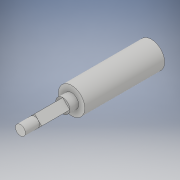
# Autodesk Inventor part: MainGearShaft
Saved by Autodesk Inventor 2017 (Build 210142000, 142)
## iProperties
Created: 2020-04-04
Part Number: MainGearShaft
Material: Generic
Document SubType Name: Modeling
Designer: LaNave
Density: 1 g/cm^3
Appearance: Default
Mass: 3.54669 g
Surface Area: 26.9064 cm^2
Volume: 3.54669 cm^3
Author: LaNave
## iProperties of the stored document gear1-shaft_3DPrint.ipt
Created: 2021-01-25
Part Number: gear1-shaft_3DPrint
Material: Generic
Document SubType Name: Modeling
Designer: agustin
Density: 1 g/cm^3
Appearance: Default
Author: agustin
Autodesk Inventor part; units mm, degrees
ref_plane "YZ Plane" through (0, 0, 0) normal (1, 0, 0) x (0, 1, 0)
ref_plane "XZ Plane" through (0, 0, 0) normal (0, 1, 0) x (-1, 0, 0)
ref_plane "XY Plane" through (0, 0, 0) normal (0, 0, 1) x (1, 0, 0)
sketch "Sketch1" plane through (0, 0, 0) normal (0, 0, 1) x (1, 0, 0)
  circle A0 centre (0, 0) radius 4.8 projected
  arc A1 (-1.2481, -4.6349) -> (4.7694, 0.541) centre (0, 0) ccw projected
  circle A2 centre (0, 0) radius 9 projected
  circle A3 centre (0, 0) radius 4.8
  circle A4 centre (0, 0) radius 7.5
  circle A5 centre (0, 0) radius 5.5
  point P0 (0, 0)
  dimension "d0" = 15
  dimension "d23" = 11
  constraints: 3 centre point, 3 coincident
  measures "d0" diameter of A4
  measures "d23" diameter of A5
extrude "Extrusion1" add sketch "Sketch1" along normal blind 9 contours A4
sketch "Sketch2" plane through (0, 0, 9) normal (0, 0, 1) x (1, 0, 0)
  line L0 (4.7694, 0.541) -> (-1.2481, -4.6349) projected
  line L1 (-4.7694, -0.541) -> (1.2481, 4.6349) projected
  circle A0 centre (0, 0) radius 7.5
  line L2 (-5.478, -0.491) -> (1.3046, 5.343)
  line L3 (-2.0867, 2.426) -> (-5.478, -0.491)
  line L4 (-1.3046, -5.343) -> (5.478, 0.491)
  line L5 (2.0867, -2.426) -> (-0.6256, -4.7591)
  arc A1 (-5.478, -0.491) -> (-1.3046, -5.343) centre (0, 0) ccw
  arc A2 (5.478, 0.491) -> (1.3046, 5.343) centre (0, 0) ccw
  constraints: 12 end point, 4 point on circle, 3 centre point, 2 midpoint, 1 coincident
extrude "Extrusion2" add sketch "Sketch2" along normal blind 34.2598
sketch "Sketch3" plane through (0, 0, 43.2598) normal (0, 0, 1) x (1, 0, 0)
  circle A0 centre (0, 0) radius 7.5 projected
  circle A1 centre (0, 0) radius 7.5
  point P0 (0, 0)
  constraints: 1 centre point, 1 coincident
extrude "Extrusion3" add sketch "Sketch3" along normal blind 2
sketch "Sketch5" plane through (0, 0, 45.2598) normal (0, 0, 1) x (1, 0, 0)
  circle A0 centre (0, 0) radius 4
  dimension "d10" = 8
  constraints: 1 centre point, 1 coincident
  measures "d10" diameter of A0
extrude "Extrusion5" add sketch "Sketch5" along normal blind 5
sketch "Sketch6" plane through (0, 0, 50.2598) normal (0, 0, 1) x (1, 0, 0)
  circle A0 centre (0, 0) radius 4 projected
  line L0 (-4, 0) -> (0, 4)
  line L1 (0, 4) -> (4, 0)
  line L2 (4, 0) -> (0, -4)
  line L3 (0, -4) -> (-4, 0)
  constraints: 8 end point, 1 horizontal alignment, 10 other
extrude "Extrusion6" add sketch "Sketch6" along normal blind 16 contours L2 L3 L0 L1
sketch "Sketch7" plane through (0, 0, 66.2598) normal (0, 0, 1) x (1, 0, 0)
  circle A0 centre (0, 0) radius 2.8284
  line L0 (0, 4) -> (-4, 0) projected
  constraints: 1 centre point, 1 coincident, 1 tangent
extrude "Extrusion7" add sketch "Sketch7" along normal blind 8
sketch "Sketch8" plane through (0, 0, 9) normal (0, 0, -1) x (-1, 0, 0)
  point P0 (0, 0)
sketch "Sketch9" plane through (0, 0, 43.2598) normal (0, 0, -1) x (-1, 0, 0)
  line L0 (1.0362, -6.2993) -> (-6.5532, 0.2287)
  line L1 (6.1416, 0.1254) -> (-2.464, 7.5275)
  arc A0 (0.1057, -5.499) -> (5.453, 0.7177) centre (0, 0) ccw
  arc A1 (-0.1057, 5.499) -> (-5.453, -0.7177) centre (0, 0) ccw
  point P0 (0, 0)
  point P1 (0, 0)
  constraints: 4 end point, 4 point on circle, 4 point on line, 2 centre point
extrude "Extrusion8" cut sketch "Sketch9" along normal blind 50
sketch "Sketch10" plane through (0, 0, 43.2598) normal (0, 0, -1) x (-1, 0, 0)
  circle A0 centre (0, 0) radius 5.5
  dimension "d28" = 11
  constraints: 1 centre point, 1 coincident
  measures "d28" diameter of A0
extrude "Extrusion9" cut sketch "Sketch10" along normal blind 50
sketch "Sketch11" plane through (0, 0, 43.2598) normal (0, 0, -1) x (-1, 0, 0)
  line L0 (-4.1828, 4.1) -> (4.1828, 4.1)
  line L1 (4.1828, -4.1) -> (-4.1828, -4.1)
  line L2 (-12.4976, 4.1) -> (12.4976, -4.1) construction
  line L3 (12.4976, 4.1) -> (-12.4976, -4.1) construction
  arc A0 (4.1828, 4.1) -> (-4.1828, 4.1) centre (0, 0) ccw
  arc A1 (-4.1828, -4.1) -> (4.1828, -4.1) centre (0, 0) ccw
  point P0 (0, 0)
  dimension "d34" = 8.2
  constraints: 8 end point, 4 point on circle, 2 centre point, 2 midpoint, 1 horizontal, 1 parallel
  measures "d34" distance between parallel lines of L1 L0
extrude "Extrusion10" add sketch "Sketch11" along normal blind 39.4125
scale "Scale1" factors (0.5, 0.5, 0.5) then translate (0, 0, 11.3149) bodies 1
body "Solid1"
